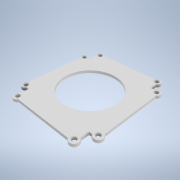
# Autodesk Inventor part: PCB Bracket 2
Saved by Autodesk Inventor 2020 (Build 240168000, 168)
## iProperties
Created: 2019-07-09
Part Number: PCB Bracket 2
Material: Generic
Document SubType Name: Modeling
Designer: anwar
Density: 1 g/cm^3
Appearance: Default
Author: anwar
Autodesk Inventor part; units mm, degrees
ref_plane "YZ Plane" through (0, 0, 0) normal (1, 0, 0) x (0, 1, 0)
ref_plane "XZ Plane" through (0, 0, 0) normal (0, 1, 0) x (-1, 0, 0)
ref_plane "XY Plane" through (0, 0, 0) normal (0, 0, 1) x (1, 0, 0)
sketch "Sketch5" plane through (0, 0, 0) normal (0, 1, 0) x (-1, 0, 0)
  line L0 (-22.9, -32.9) -> (22.9, 32.9) construction
  line L1 (22.9, -32.9) -> (-22.9, 32.9) construction
  circle A0 centre (22.9, 32.9) radius 1.5
  circle A1 centre (22.9, -32.9) radius 1.5
  circle A2 centre (-22.9, 32.9) radius 1.5
  circle A3 centre (-22.9, -32.9) radius 1.5
  point P0 (0, 0)
  dimension "d6" = 45.8
  dimension "d7" = 65.8
  dimension "d8" = 3
  dimension "d9" = 3
  dimension "d10" = 3
  dimension "d11" = 3
  constraints: 4 centre point, 4 coincident, 4 end point, 2 midpoint
  measures "d6" distance of L1.end L0.end
  measures "d7" distance of L0.end L1.start
  measures "d8" diameter of A0
  measures "d9" diameter of A1
  measures "d10" diameter of A2
  measures "d11" diameter of A3
sketch "Sketch8" plane through (0, 0, 0) normal (0, 1, 0) x (-1, 0, 0)
  line L0 (28.9, -23.5) -> (-28.9, 23.5) construction
  line L1 (-28.9, -23.5) -> (28.9, 23.5) construction
  circle A0 centre (28.9, 23.5) radius 1.5
  circle A1 centre (28.9, -23.5) radius 1.5
  circle A2 centre (-28.9, 23.5) radius 1.5
  circle A3 centre (-28.9, -23.5) radius 1.5
  point P0 (0, 0)
  dimension "d24" = 57.8
  dimension "d25" = 47
  dimension "d26" = 3
  dimension "d27" = 3
  dimension "d28" = 3
  dimension "d29" = 3
  constraints: 4 centre point, 4 end point, 3 coincident, 2 midpoint
  measures "d24" distance of L0.end L1.end
  measures "d25" distance of L1.start L0.end
  measures "d26" diameter of A0
  measures "d27" diameter of A1
  measures "d28" diameter of A2
  measures "d29" diameter of A3
sketch "Sketch10" plane through (0, 0, 0) normal (0, 1, 0) x (-1, 0, 0)
  line L0 (-24.4, -34.4) -> (24.4, -34.4)
  line L1 (24.4, -34.4) -> (24.4, 34.4)
  line L2 (24.4, 34.4) -> (-24.4, 34.4)
  line L3 (-24.4, 34.4) -> (-24.4, -34.4)
  line L4 (-24.4, -34.4) -> (24.4, 34.4) construction
  line L5 (24.4, -34.4) -> (-24.4, 34.4) construction
  line L6 (-30.4, -25) -> (30.4, -25)
  line L7 (30.4, -25) -> (30.4, 25)
  line L8 (30.4, 25) -> (-30.4, 25)
  line L9 (-30.4, 25) -> (-30.4, -25)
  line L10 (-30.4, -25) -> (30.4, 25) construction
  line L11 (30.4, -25) -> (-30.4, 25) construction
  circle A0 centre (28.8992, 23.4996) radius 3
  circle A1 centre (22.8996, 32.8995) radius 3
  circle A2 centre (28.8992, -23.4965) radius 3
  circle A3 centre (22.8996, -32.9046) radius 3
  circle A4 centre (-28.9017, -23.4965) radius 3
  circle A5 centre (-22.8972, -32.9046) radius 3
  circle A6 centre (-28.9017, 23.4996) radius 3
  circle A7 centre (-22.8972, 32.8995) radius 3
  point P0 (0, 0)
  point P1 (24.4, 25)
  point P2 (24.4, 30.3016)
  point P3 (20.3018, 34.4)
  point P4 (-20.2994, 34.4)
  point P5 (-24.4, 30.303)
  point P6 (-24.4, 25)
  point P7 (-26.3038, 25)
  point P8 (-30.4, 20.9006)
  point P9 (-30.4, -20.8974)
  point P10 (-26.3056, -25)
  point P11 (-24.4, -25)
  point P12 (-24.4, -30.3081)
  point P13 (-20.2965, -34.4)
  point P14 (20.2989, -34.4)
  point P15 (24.4, -30.3067)
  point P16 (24.4, -25)
  point P17 (26.3031, -25)
  point P18 (30.4, -20.8989)
  point P19 (30.4, 20.902)
  point P20 (26.3013, 25)
  dimension "d46" = 48.8
  dimension "d47" = 68.8
  dimension "d48" = 60.8
  dimension "d49" = 50
  dimension "d50" = 6
  dimension "d51" = 6
  dimension "d52" = 6
  dimension "d53" = 6
  dimension "d54" = 6
  dimension "d55" = 6
  dimension "d56" = 6
  dimension "d57" = 6
  constraints: 24 end point, 8 centre point, 4 midpoint, 4 parallel, 2 horizontal, 2 perpendicular
  measures "d46" distance of L2.end L1.end
  measures "d47" distance of L1.end L0.end
  measures "d48" distance of L8.end L7.end
  measures "d49" distance of L7.end L6.end
  measures "d50" diameter of A0
  measures "d51" diameter of A1
  measures "d52" diameter of A2
  measures "d53" diameter of A3
  measures "d54" diameter of A4
  measures "d55" diameter of A5
  measures "d56" diameter of A6
  measures "d57" diameter of A7
extrude "Extrusion3" add sketch "Sketch10" along normal blind 2
extrude "Extrusion4" cut sketch "Sketch5" along normal blind 2
extrude "Extrusion5" cut sketch "Sketch8" along normal blind 2
sketch "Sketch11" plane through (0, 2, 0) normal (0, 1, 0) x (1, 0, 0)
  circle A0 centre (0, 0) radius 20
  dimension "d64" = 40
  constraints: 1 centre point, 1 coincident
  measures "d64" diameter of A0
extrude "Extrusion6" cut sketch "Sketch11" against normal blind 2
body "Solid2"
